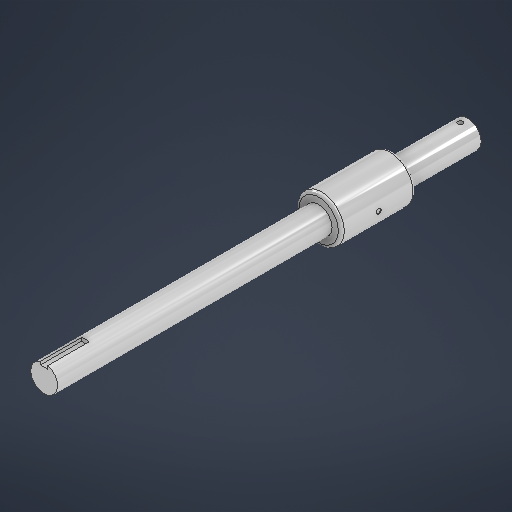
# Autodesk Inventor part: Final joint shaft
Saved by Autodesk Inventor 2026.3 (Build 303398000, 398)
## iProperties
Created: 2026-08-01
Part Number: Final joint shaft
Material: Generic
Document SubType Name: Sheet Metal
Designer: matot
Density: 1 g/cm^3
Sheet Metal Rule: Default_mm
Appearance: Default
Author: matot
Autodesk Inventor part; units mm, degrees
ref_plane "YZ Plane" through (0, 0, 0) normal (1, 0, 0) x (0, 1, 0)
ref_plane "XZ Plane" through (0, 0, 0) normal (0, 1, 0) x (-1, 0, 0)
ref_plane "XY Plane" through (0, 0, 0) normal (0, 0, 1) x (1, 0, 0)
sketch "Sketch1" plane through (0, 0, 0) normal (0, 0, 1) x (1, 0, 0)
  circle A0 centre (0, 0) radius 15.25
  dimension "d0" = 30.5
  constraints: 1 centre point, 1 coincident
  measures "d0" diameter of A0
extrude "Extrusion1" add sketch "Sketch1" along normal blind 50
fillet "Fillet1" radius 2 1 edges at (-15.25, 0, 50)
fillet "Fillet2" radius 2 1 edges at (-15.25, 0, 0)
sketch "Sketch2" plane through (0, 0, 50) normal (0, 0, 1) x (1, 0, 0)
  circle A0 centre (0, 0) radius 9
  dimension "d5" = 18
  constraints: 1 centre point, 1 coincident
  measures "d5" diameter of A0
extrude "Extrusion2" add sketch "Sketch2" along normal blind 184
sketch "Sketch3" plane through (0, 0, 0) normal (0, 0, -1) x (-1, 0, 0)
  circle A0 centre (0, 0) radius 9
  constraints: 1 centre point, 1 coincident
extrude "Extrusion3" add sketch "Sketch3" along normal blind 50
sketch "Sketch4" plane through (0, 0, -50) normal (0, 0, -1) x (-1, 0, 0)
  circle A0 centre (0, 0) radius 3
  dimension "d10" = 6
  constraints: 1 centre point, 1 coincident
  measures "d10" diameter of A0
extrude "Extrusion4" cut sketch "Sketch4" against normal blind 13
sketch "Sketch5" plane through (0, 0, -50) normal (0, 0, -1) x (-1, 0, 0)
  circle A0 centre (0, 0) radius 9 projected
  point P0 (0, 9)
  constraints: 1 vertical alignment, 1 other
ref_plane "Work Plane1" through (0, 9, -50) normal (0, 1, 0) x (-1, 0, 0)
sketch "Sketch6" plane through (0, 9, -50) normal (0, 1, 0) x (-1, 0, 0)
  line L0 (-9, 0) -> (9, 0) projected
  point P0 (0, 50)
  point P1 (0, 5)
  dimension "d13" = 5
  measures "d13" distance from line of L0 point (0, 5)
hole "Hole1" at (0, 9, -45) direction (0, -1, 0) diameter 3.242 depth 9 tip angle 118 thread size "M4x0.7" class "6H" standard "ISO Metric profile"
sketch "Sketch7" plane through (0, 0, 0) normal (0, 0, -1) x (-1, 0, 0)
  circle A0 centre (0, 0) radius 15.25 projected
  point P0 (-15.25, 0)
  constraints: 1 horizontal alignment, 1 other
ref_plane "Work Plane2" through (15.25, 0, 0) normal (1, 0, 0) x (0, 1, 0)
sketch "Sketch8" plane through (15.25, 0, 0) normal (1, 0, 0) x (0, 1, 0)
  point P0 (0, 0)
  point P1 (0, 25)
  dimension "d21" = 25
  measures "d21" distance of point (0, 25) point (0, 0)
hole "Hole2" at (15.25, 0, 25) direction (-1, 0, 0) diameter 3.242 depth 0.5 tip angle 118 thread size "M4x0.7" class "6H" standard "ISO Metric profile"
sketch "Sketch9" plane through (0, 0, 234) normal (0, 0, 1) x (1, 0, 0)
  circle A0 centre (0, 0) radius 9 projected
  line L0 (2.5, 8.9) -> (2.5, 6.5)
  line L1 (2.5, 6.5) -> (-2.5, 6.5)
  line L2 (-2.5, 6.5) -> (-2.5, 8.6458)
  line L3 (-2.5, 6.5) -> (-2.5, 9)
  line L4 (-2.5, 9) -> (2.5, 9)
  line L5 (2.5, 9) -> (2.5, 6.8873)
  line L6 (-2.5, 9) -> (-2.5, 6.5)
  line L7 (-2.5, 6.5) -> (2.5, 6.5)
  point P0 (0, 6.5)
  point P1 (2.5, 7.7)
  point P2 (2.5, 8.6458)
  dimension "d29" = 5
  dimension "d31" = 0
  dimension "d32" = 2.5
  dimension "d33" = 6.5
  dimension "d34" = 2.5
  constraints: 16 end point, 2 collinear, 2 midpoint, 1 parallel, 1 perpendicular, 1 point on line, 1 vertical, 2 other
  measures "d29" distance of L0.end L1.end
  measures "d31" horizontal distance of point (0, 0) point (0, 6.5)
  measures "d32" distance between parallel lines of L1 L4
  measures "d33" distance from line of point (0, 0) L1
  measures "d34" horizontal distance of point (2.5, 7.7) point (0, 6.5)
extrude "Extrusion5" cut sketch "Sketch9" against normal blind 27.5 contours A0 L0 L1 L2 picked at (0, 7.3333)
equation "\"d27\" = Thickness"
equation "\"BendRadius\" = Thickness"
equation "\"BendReliefWidth\" = Thickness"
equation "\"BendReliefDepth\" = 0.5 * Thickness"
equation "\"CornerReliefSize\" = 4 * Thickness"
equation "\"MinimumRemnant\" = 2 * Thickness"
equation "\"TransitionRadius\" = BendRadius"
equation "\"JacobiRadiusSize\" = BendRadius"
equation "\"GapSize\" = Thickness"
equation "\"Thickness\" = 0.5"
body "Solid1"
